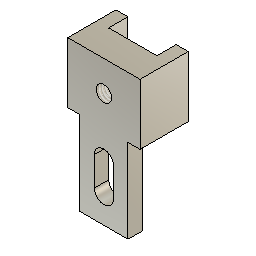
Slider (Autodesk Fusion 360 design; units mm, degrees)
Autodesk Fusion 360 part; units mm, degrees
sketch "Sketch1" plane through (0, 0, 0) normal (0, 1, 0) x (1, 0, 0) in component "Slider"
  line L0 (9.525, 8) -> (-9.525, 8)
  line L1 (9.525, -8) -> (9.525, 8)
  line L2 (-9.525, -8) -> (9.525, -8)
  line L3 (-9.525, 8) -> (-9.525, -8)
  line L4 (-6.35, 30.1) -> (-6.35, -8)
  line L5 (6.35, 30.1) -> (-6.35, 30.1)
  line L6 (6.35, -8) -> (6.35, 30.1)
  line L7 (-2.54, 22.86) -> (-2.54, 15.24)
  arc A0 (-2.54, 15.24) -> (2.54, 15.24) centre (0, 15.24) ccw
  line L8 (2.54, 15.24) -> (2.54, 22.86)
  arc A1 (2.54, 22.86) -> (-2.54, 22.86) centre (0, 22.86) ccw
  line L9 (0, 25.4) -> (0, 12.7) construction
  circle A2 centre (0, 0) radius 1.8987
  circle A3 centre (0, 0) radius 3.175
  circle A4 centre (0, 0) radius 12.7 construction
  circle A5 centre (0, 15.24) radius 3.9624 construction
  circle A6 centre (0, 22.86) radius 3.9624 construction
  point P0 (0, 0)
  dimension "d2_1" = 5.08
  dimension "d4_1" = 6.35
  dimension "d5_1" = 3.7973
  dimension "d9_1" = 19.05
  dimension "d10_1" = 6.35
  dimension "d12_1" = 6.35
  dimension "d15_1" = 15.24
  dimension "d16_1" = 12.7
  dimension "d19_1" = 9.525
  dimension "d50_1" = 8
  dimension "d51_1" = 8
  dimension "d52_1" = 25.4
  dimension "d53_1" = 7.9248
  dimension "d54_1" = 7.9248
  dimension "d55_1" = 38.1
  constraint coincident L2 L6.start
  constraint coincident L2 L4.end
  constraint tangent L7 A0
  constraint tangent A0 L8
  constraint parallel L7 L8
  constraint tangent L8 A1
  constraint tangent L7 A1
  constraint midpoint A1 L9.start
  constraint midpoint A0 L9.end
  constraint parallel L4 L9
  constraint concentric A2 A3
  constraint coincident P0 A2.centre
  constraint horizontal L2
  constraint vertical L4
  constraint vertical L6
  constraint vertical L3
  constraint vertical L1
  constraint horizontal L5
  constraint vertical A0.centre P0
  constraint concentric A2 A4
  constraint concentric A0 A5
  constraint concentric A1 A6
  constraint horizontal L0
  measures "d2_1" diameter of A0
  measures "d4_1" diameter of A3
  measures "d5_1" diameter of A2
  measures "d9_1" distance of L1.start L2.start
  measures "d10_1" distance of L4 P0
  measures "d12_1" distance of L6 P0
  measures "d15_1" distance of A0.centre P0
  measures "d16_1" distance of L9.start L9.end
  measures "d19_1" distance of L1 P0
  measures "d50_1" distance of L2 P0
  measures "d51_1" distance of L0 P0
  measures "d52_1" diameter of A4
  measures "d53_1" diameter of A5
  measures "d54_1" diameter of A6
  measures "d55_1" distance of L4.start L4.end
extrude "Extrude1" add sketch "Sketch1" along normal blind 3.81 contours L0 L2 L4 L6 | L0 L4 L5 L6 in component "Slider"
extrude "Extrude2" add sketch "Sketch1" along normal blind 7.62 contours L0 L2 L4 L6 | A3 in component "Slider"
extrude "Extrude3" add sketch "Sketch1" along normal blind 12.7 contours L0 L1 L2 L6 | L0 L2 L3 L4 in component "Slider"
thread "Thread1" "ANSI Unified Screw Threads 0.19(#10) 10-32 UNF 3B" major diameter 4.826 minor diameter 4.0665 pitch 0.7937 angle 60 resizes the face on face at (1.8963, 5.08, 0.0946) in component "Slider"
component "Slider" placed x (1, 0, 0) y (0, 1, 0) z (0, 0, 1) at (0, 0, 0)
equation "d12_1 = d10_1"
equation "d53_1 = ( 3.9624 * 2 ) * 1 mm"
equation "d54_1 = d53_1"
